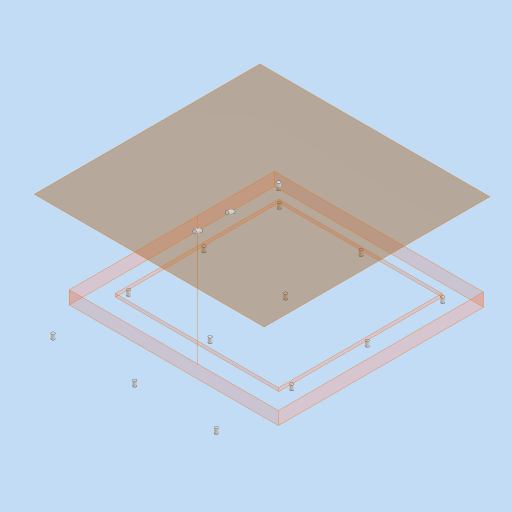
# Autodesk Inventor part: HF-Kabelführung-V2-XGantry-LängenSkizze
Saved by Autodesk Inventor 2023.2 (Build 272271000, 271)
## iProperties
Created: 2023-12-13
Part Number: HF-Kabelführung-V2-XGantry-LängenSkizze
Material: Generisch
Document SubType Name: Modeling
Designer: Nils Bade
Density: 1 g/cm^3
Appearance: Vorgabe
Author: Nils Bade
Autodesk Inventor part; units mm, degrees
ref_plane "YZ Plane" through (0, 0, 0) normal (1, 0, 0) x (0, 1, 0)
ref_plane "XY Plane" through (0, 0, 0) normal (0, 0, 1) x (1, 0, 0)
sketch "S-Orientierung" plane through (0, 0, 0) normal (0, 1, 0) x (-1, 0, 0)
  line L0 (250, 0) -> (-250, 0)
  line L1 (-250, 0) -> (-250, -500)
  line L2 (-250, -500) -> (250, -500)
  line L3 (250, -500) -> (250, 0)
  line L4 (0, -691.3667) -> (0, 249.2) construction
  line L5 (-448, 0) -> (448, 0) construction
  line L6 (320, 71) -> (-320, 71)
  line L7 (-320, 71) -> (-320, -557)
  line L8 (-320, -557) -> (320, -557)
  line L9 (320, -557) -> (320, 71)
  point P0 (0, 0)
  dimension "d0" = 500
  dimension "d1" = 500
  dimension "d2" = 640
  dimension "d3" = 628
  dimension "d4" = 71
  constraints: 16 end point, 4 parallel, 2 horizontal, 2 perpendicular, 1 collinear, 2 other
  measures "d0" distance of L0.start L0.end
  measures "d1" distance of L0.end L1.end
  measures "d2" distance of L6.start L6.end
  measures "d3" distance of L6.end L7.end
  measures "d4" distance between parallel lines of L6 L0
surface extrude "Ex-AußenRahmen-AUT-Platte" sketch "S-Orientierung" along normal blind 10 shown yes curves L0 L1 L2 L3
surface extrude "Ex-Innenseiten-4040-Profile" sketch "S-Orientierung" along normal mid plane 40 shown yes curves L6 L7 L8 L9
ref_plane "Deckenebene" through (0, 295, 0) normal (0, 1, 0) x (-1, 0, 0)
sketch "S-Kabelziele" plane through (0, 0, 0) normal (0, 1, 0) x (-1, 0, 0)
  line L0 (250, 0) -> (-250, 0) projected
  line L1 (-250, 0) -> (-250, -500) projected
  line L2 (-250, -500) -> (250, -500) projected
  line L3 (250, -500) -> (250, 0) projected
  line L4 (320, 71) -> (-320, 71) projected
  line L5 (-290, 25) -> (290, 25) construction
  line L6 (-290, -517) -> (290, -517) construction
  line L7 (320, -557) -> (-320, -557) construction
  line L8 (-290, -557) -> (-290, 71) construction
  line L9 (290, -557) -> (290, 71) construction
  line L10 (320, 71) -> (320, -557) construction
  line L11 (-320, -557) -> (-320, 71) construction
  line L12 (-210, -55) -> (-290, -55)
  line L13 (-290, -55) -> (-290, 25)
  line L14 (-290, 25) -> (-210, 25)
  line L15 (-210, 25) -> (-210, -55)
  line L16 (-210, -55) -> (-290, 25) construction
  line L17 (-290, -55) -> (-210, 25) construction
  line L18 (-250, -55) -> (-250, 25) construction
  circle A0 centre (-250, -40) radius 5
  line L19 (-210, -517) -> (-290, -517)
  line L20 (-290, -517) -> (-290, -437)
  line L21 (-290, -437) -> (-210, -437)
  line L22 (-210, -437) -> (-210, -517)
  line L23 (-210, -517) -> (-290, -437) construction
  line L24 (-290, -517) -> (-210, -437) construction
  line L25 (-250, -517) -> (-250, -437) construction
  circle A1 centre (-250, -502) radius 5
  line L26 (290, -517) -> (210, -517)
  line L27 (210, -517) -> (210, -437)
  line L28 (210, -437) -> (290, -437)
  line L29 (290, -437) -> (290, -517)
  line L30 (290, -517) -> (210, -437) construction
  line L31 (210, -517) -> (290, -437) construction
  line L32 (250, -517) -> (250, -437) construction
  circle A2 centre (250, -502) radius 5
  line L33 (290, -55) -> (210, -55)
  line L34 (210, -55) -> (210, 25)
  line L35 (210, 25) -> (290, 25)
  line L36 (290, 25) -> (290, -55)
  line L37 (290, -55) -> (210, 25) construction
  line L38 (210, -55) -> (290, 25) construction
  line L39 (250, -55) -> (250, 25) construction
  circle A3 centre (250, -40) radius 5
  line L40 (40, -55) -> (-40, -55)
  line L41 (-40, -55) -> (-40, 25)
  line L42 (-40, 25) -> (40, 25)
  line L43 (40, 25) -> (40, -55)
  line L44 (40, -55) -> (-40, 25) construction
  line L45 (-40, -55) -> (40, 25) construction
  line L46 (0, -55) -> (0, 25) construction
  circle A4 centre (0, -40) radius 5
  line L47 (40, -517) -> (-40, -517)
  line L48 (-40, -517) -> (-40, -437)
  line L49 (-40, -437) -> (40, -437)
  line L50 (40, -437) -> (40, -517)
  line L51 (40, -517) -> (-40, -437) construction
  line L52 (-40, -517) -> (40, -437) construction
  line L53 (0, -517) -> (0, -437) construction
  circle A5 centre (0, -502) radius 5
  line L54 (0, -638.7667) -> (0, 240.4333) construction
  point P0 (0, 0)
  point P1 (-250, -15)
  point P2 (-250, -477)
  point P3 (250, -477)
  point P4 (250, -15)
  point P5 (0, -15)
  point P6 (0, -477)
  point P7 (0, -477)
  point P8 (0, -15)
  dimension "d10" = 46
  dimension "d11" = 40
  dimension "d12" = 30
  dimension "d13" = 30
  dimension "d14" = 80
  dimension "d15" = 80
  dimension "d16" = 10
  dimension "d18" = 65
  dimension "d19" = 80
  dimension "d20" = 80
  dimension "d21" = 10
  dimension "d22" = 65
  dimension "d23" = 80
  dimension "d24" = 80
  dimension "d25" = 10
  dimension "d26" = 65
  dimension "d27" = 80
  dimension "d28" = 80
  dimension "d29" = 10
  dimension "d30" = 65
  dimension "d31" = 80
  dimension "d32" = 80
  dimension "d33" = 10
  dimension "d34" = 65
  dimension "d35" = 80
  dimension "d36" = 80
  dimension "d37" = 10
  dimension "d38" = 65
  constraints: 92 end point, 26 midpoint, 14 point on line, 12 parallel, 10 collinear, 8 horizontal, 6 centre point, 6 perpendicular, 2 vertical, 3 other
  measures "d10" distance between parallel lines of L4 L5
  measures "d11" distance between parallel lines of L6 L7
  measures "d12" distance between parallel lines of L8 L11
  measures "d13" distance between parallel lines of L10 L9
  measures "d14" distance of L13.end L14.end
  measures "d15" distance of L12.end L13.end
  measures "d16" diameter of A0
  measures "d18" distance from line of L14 A0.centre
  measures "d19" distance of L20.end L21.end
  measures "d20" distance of L20.start L20.end
  measures "d21" diameter of A1
  measures "d22" distance from line of L21 A1.centre
  measures "d23" distance of L27.end L28.end
  measures "d24" distance of L27.start L27.end
  measures "d25" diameter of A2
  measures "d26" distance from line of L28 A2.centre
  measures "d27" distance of L34.end L35.end
  measures "d28" distance of L34.start L34.end
  measures "d29" diameter of A3
  measures "d30" distance from line of L35 A3.centre
  measures "d31" distance of L41.end L42.end
  measures "d32" distance of L41.start L41.end
  measures "d33" diameter of A4
  measures "d34" distance from line of L42 A4.centre
  measures "d35" distance of L48.end L49.end
  measures "d36" distance of L48.start L48.end
  measures "d37" diameter of A5
  measures "d38" distance from line of L49 A5.centre
sketch "S-FeedIn-Points" plane through (0, 0, 0) normal (1, 0, 0) x (0, 1, 0)
  line L0 (295, 196.6) -> (295, -682.6) construction
  line L1 (-627.6561, 0) -> (627.6561, 0) construction
  line L2 (307.8171, 5.9767) -> (298.4202, 9.3969)
  line L3 (298.4202, 9.3969) -> (291.5798, -9.3969)
  line L4 (291.5798, -9.3969) -> (300.9767, -12.8171)
  line L5 (300.9767, -12.8171) -> (307.8171, 5.9767)
  line L6 (0, -500) -> (10, -500) projected
  line L7 (0, -500) -> (295, -500)
  line L8 (295, -500) -> (295, 0)
  line L9 (295, 0) -> (0, 0)
  line L10 (0, 0) -> (0, -500)
  line L11 (305, -245) -> (285, -245)
  line L12 (285, -245) -> (285, -255)
  line L13 (285, -255) -> (305, -255)
  line L14 (305, -255) -> (305, -245)
  line L15 (305, -245) -> (285, -255) construction
  line L16 (285, -245) -> (305, -255) construction
  point P0 (295, -250)
  dimension "d46" = 20
  dimension "d47" = 10
  dimension "d48" = 20
  dimension "d55" = 20
  dimension "d56" = 10
  constraints: 28 end point, 6 parallel, 4 midpoint, 4 perpendicular, 2 point on line, 1 horizontal
  measures "d46" distance between parallel lines of L2 L4
  measures "d47" distance between parallel lines of L3 L5
  measures "d48" angle of L0 L3
  measures "d55" distance of L11.start L11.end
  measures "d56" distance of L12.end L11.end
extrude "Ex-FeedIn1-1" add sketch "S-FeedIn-Points" along normal mid plane 10 contours L5 L4 L8 L3 L2 | L8 L4 L3
sketch "Skizze5" plane through (-5, 298.4202, 9.3969) normal (0, 0.3420201, 0.9396926) x (1, 0, 0)
  line L0 (10, 0) -> (0, 0) projected
  line L1 (10, 10) -> (10, 0) projected
  line L2 (0, 10) -> (10, 10) projected
  line L3 (0, 0) -> (0, 10) projected
  circle A0 centre (5, 5) radius 5
  line L4 (10, 0) -> (10, 10) projected
  point P0 (5, -277.2093)
  point P1 (0, 5)
  point P2 (5, 10)
  point P3 (10, 5)
  point P4 (5, 0)
  constraints: 1 centre point, 1 tangent
extrude "Ex-FeedIn1-2" cut sketch "Skizze5" against normal up to surface (20 mm away) contours L0 A0 L1 | L0 L3 A0 | A0 L2 L1 | L3 L2 A0
extrude "Ex-FeedOut" add sketch "S-Kabelziele" against normal blind 15 separate body contours A3 L3 | L3 A3 | A2 L2 L3 | L3 L2 A2 | A0 L1 | L1 A0 | A1 L2 L1 | L1 L2 A1 | A5 L2 | L2 A5 | A4
extrude "Ex-FeedIn2-1" add sketch "S-FeedIn-Points" along normal mid plane 10 separate body contours L11 L14 L13 L8 | L8 L13 L12 L11
sketch "Skizze6" plane through (-5, 305, -245) normal (0, 1, 0) x (1, 0, 0)
  line L0 (10, 0) -> (0, 0) projected
  line L1 (10, 10) -> (10, 0) projected
  line L2 (0, 10) -> (10, 10) projected
  line L3 (0, 0) -> (0, 10) projected
  circle A0 centre (5, 5) radius 5
  line L4 (0, 10) -> (10, 10) projected
  point P0 (5, -245)
  point P1 (0, 5)
  point P2 (5, 10)
  point P3 (10, 5)
  point P4 (5, 0)
  constraints: 1 centre point, 1 tangent
extrude "Ex-FeedIn2-2" cut sketch "Skizze6" against normal up to surface (20 mm away) contours L0 A0 L1 | L0 L3 A0 | A0 L2 L1 | L3 L2 A0 bodies 3
pattern_linear "Rechteckige Anordnung1" count 2 spacing 100 along (0, 0, -1) bodies 1
pattern_linear "Rechteckige Anordnung2" count 2 spacing 231 along (0, 0, 1) of "Ex-FeedOut" bodies 2
equation "\"d18\" = d30"
equation "\"d22\" = d30"
equation "\"d26\" = d30"
equation "\"d34\" = d30"
equation "\"d38\" = d30"
